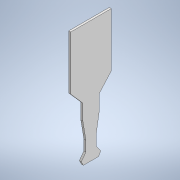
# Autodesk Inventor part: support_board_3
Saved by Autodesk Inventor 2020 (Build 240168000, 168)
## iProperties
Created: 2019-05-15
Part Number: support_board_3
Material: Generic
Document SubType Name: Modeling
Designer: psrob
Density: 1 g/cm^3
Appearance: Default
Author: psrob
Autodesk Inventor part; units mm, degrees
ref_plane "YZ Plane" through (0, 0, 0) normal (1, 0, 0) x (0, 1, 0)
ref_plane "XZ Plane" through (0, 0, 0) normal (0, 1, 0) x (-1, 0, 0)
ref_plane "XY Plane" through (0, 0, 0) normal (0, 0, 1) x (1, 0, 0)
sketch "Sketch1" plane through (0, 0, 0) normal (1, 0, 0) x (0, 1, 0)
  line L0 (0, -13) -> (3, -16) projected
  line L1 (18.4, -16) -> (3, -16) projected
  line L2 (32, -27.9999) -> (18.4, -16) projected
  line L3 (40, -27.9999) -> (32, -27.9999) projected
  line L4 (40, -27.9999) -> (40, -8) projected
  line L5 (40, -8) -> (0, -8) projected
  line L6 (0, -13) -> (0, -8) projected
  line L7 (0, -3) -> (3, 0) projected
  line L8 (0, -3) -> (0, -8) projected
  line L9 (40, -8) -> (0, -8) projected
  line L10 (40, 12) -> (40, -8) projected
  line L11 (40, 12) -> (32, 12) projected
  line L12 (32, 12) -> (18.4, 0) projected
  line L13 (18.4, 0) -> (3, 0) projected
  line L14 (-54.8834, 12) -> (-44.8834, 2) projected
  line L15 (-44.8834, 2) -> (-44.8834, -8) projected
  line L16 (-44.8834, -8) -> (-14.8834, -8) projected
  line L17 (-14.8834, -3) -> (-14.8834, -8) projected
  line L18 (-24.8834, -3) -> (-14.8834, -3) projected
  line L19 (-24.8834, -3) -> (-44.8834, 12) projected
  line L20 (-54.8834, 12) -> (-44.8834, 12) projected
  line L21 (-54.8834, -28) -> (-44.8834, -18) projected
  line L22 (-54.8834, -28) -> (-44.8834, -28) projected
  line L23 (-24.8834, -13) -> (-44.8834, -28) projected
  line L24 (-24.8834, -13) -> (-14.8834, -13) projected
  line L25 (-14.8834, -13) -> (-14.8834, -8) projected
  line L26 (-44.8834, -8) -> (-14.8834, -8) projected
  line L27 (-44.8834, -18) -> (-44.8834, -8) projected
  line L28 (-34.8834, -20.5) -> (-34.8834, 4.5) projected
  line L29 (-14.8834, -3) -> (3, 0)
  line L30 (-14.8834, -13) -> (3, -16)
  line L31 (40, 12) -> (55, 12)
  line L32 (55, 12) -> (55, -28)
  line L33 (55, -28) -> (40, -28)
  line L34 (40, -28) -> (40, 12)
  point P0 (0, 0)
  dimension "d0" = 15
  dimension "d1" = 40
  constraints: 12 end point, 2 parallel, 1 horizontal, 1 perpendicular
  measures "d0" distance of L32.end L33.end
  measures "d1" distance of L31.end L32.end
extrude "Extrusion1" add sketch "Sketch1" along normal blind 2 contours L6 L5 L4 L3 L2 L1 L0 | L0 L30 L25 L17 L29 L7 L8 L6 | L8 L7 L13 L12 L11 L10 L5 | L24 L23 L28 L16 L25 | L10 L31 L32 L33 L4 | L16 L28 L19 L18 L17
chamfer "Chamfer1" distance 5 angle 45 2 edges at (1, -34.8834, 4.5) (1, -34.8834, -20.5)
sketch "Sketch2" plane through (0, 0, 0) normal (-1, 0, 0) x (0, 0, 1)
  line L0 (-15.5, -34.8834) -> (-17.5, -30.8834) projected
  line L1 (-0.5, -34.8834) -> (-15.5, -34.8834) projected
  line L2 (1.5, -30.8834) -> (-0.5, -34.8834) projected
  line L3 (-3, -24.8834) -> (1.5, -30.8834) projected
  line L4 (-3, -14.8834) -> (-3, -24.8834) projected
  line L5 (0, 3) -> (-3, -14.8834) projected
  line L6 (0, 18.4) -> (0, 3) projected
  line L7 (12, 32) -> (0, 18.4) projected
  line L8 (12, 55) -> (12, 32) projected
  line L9 (-28, 55) -> (12, 55) projected
  line L10 (-28, 40) -> (-28, 55) projected
  line L11 (-27.9999, 40) -> (-28, 40) projected
  line L12 (-27.9999, 32) -> (-27.9999, 40) projected
  line L13 (-16, 18.4) -> (-27.9999, 32) projected
  line L14 (-16, 3) -> (-16, 18.4) projected
  line L15 (-13, -14.8834) -> (-16, 3) projected
  line L16 (-13, -24.8834) -> (-13, -14.8834) projected
  line L17 (-17.5, -30.8834) -> (-13, -24.8834) projected
  line L18 (-28, 55) -> (12, 55) projected
  line L19 (12, 55) -> (-28, 55)
  line L20 (-28, 55) -> (-28, 85)
  line L21 (-28, 85) -> (12, 85)
  line L22 (12, 85) -> (12, 55)
  point P0 (0, 0)
  dimension "d7" = 40
  dimension "d8" = 30
  constraints: 8 end point, 2 parallel, 1 horizontal, 1 perpendicular
  measures "d7" distance of L20.end L21.end
  measures "d8" distance of L19.end L20.end
extrude "Extrusion2" add sketch "Sketch2" against normal blind 2 contours L20 L21 L22 L9
body "Solid1"
